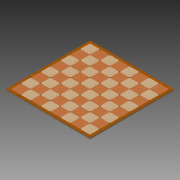
# Autodesk Inventor part: Spielfeld
Saved by Autodesk Inventor 2013 SP1 (Build 170176100, 176)
## iProperties
Created: 2012-12-06
Part Number: Spielfeld
Material: Esche
Document SubType Name: Modeling
Designer: Sebastian
Density: 1 g/cm^3
Author: Sebastian
Autodesk Inventor part; units mm, degrees
ref_plane "YZ Plane" through (0, 0, 0) normal (1, 0, 0) x (0, 1, 0)
ref_plane "XZ Plane" through (0, 0, 0) normal (0, 1, 0) x (-1, 0, 0)
ref_plane "XY Plane" through (0, 0, 0) normal (0, 0, 1) x (1, 0, 0)
sketch "Skizze5" plane through (0, 0, 0) normal (0, 0, 1) x (1, 0, 0)
  line L0 (0, 0) -> (40, 0)
  line L1 (40, 0) -> (40, 40)
  line L2 (40, 40) -> (0, 40)
  line L3 (0, 40) -> (0, 0)
  line L4 (40, 40) -> (80, 40)
  line L5 (80, 40) -> (80, 80)
  line L6 (80, 80) -> (40, 80)
  line L7 (40, 80) -> (40, 40)
  line L8 (80, 40) -> (120, 40)
  line L9 (120, 40) -> (120, 0)
  line L10 (120, 0) -> (80, 0)
  line L11 (80, 0) -> (80, 40)
  line L12 (120, 40) -> (160, 40)
  line L13 (160, 40) -> (160, 80)
  line L14 (160, 80) -> (120, 80)
  line L15 (120, 80) -> (120, 40)
  line L16 (0, 40) -> (-40, 40)
  line L17 (-40, 40) -> (-40, 80)
  line L18 (-40, 80) -> (0, 80)
  line L19 (0, 80) -> (0, 40)
  line L20 (-40, 40) -> (-80, 40)
  line L21 (-80, 40) -> (-80, 0)
  line L22 (-80, 0) -> (-40, 0)
  line L23 (-40, 0) -> (-40, 40)
  line L24 (-80, 40) -> (-120, 40)
  line L25 (-120, 40) -> (-120, 80)
  line L26 (-120, 80) -> (-80, 80)
  line L27 (-80, 80) -> (-80, 40)
  line L28 (-120, 40) -> (-160, 40)
  line L29 (-160, 40) -> (-160, 0)
  line L30 (-160, 0) -> (-120, 0)
  line L31 (-120, 0) -> (-120, 40)
  line L32 (0, 80) -> (40, 80)
  line L33 (40, 80) -> (40, 120)
  line L34 (40, 120) -> (0, 120)
  line L35 (0, 120) -> (0, 80)
  line L36 (40, 120) -> (80, 120)
  line L37 (80, 120) -> (80, 160)
  line L38 (80, 160) -> (40, 160)
  line L39 (40, 160) -> (40, 120)
  line L40 (80, 120) -> (120, 120)
  line L41 (120, 120) -> (120, 80)
  line L42 (120, 80) -> (80, 80)
  line L43 (80, 80) -> (80, 120)
  line L44 (120, 120) -> (160, 120)
  line L45 (160, 120) -> (160, 160)
  line L46 (160, 160) -> (120, 160)
  line L47 (120, 160) -> (120, 120)
  line L48 (0, 120) -> (-40, 120)
  line L49 (-40, 120) -> (-40, 160)
  line L50 (-40, 160) -> (0, 160)
  line L51 (0, 160) -> (0, 120)
  line L52 (-40, 120) -> (-80, 120)
  line L53 (-80, 120) -> (-80, 80)
  line L54 (-80, 80) -> (-40, 80)
  line L55 (-40, 80) -> (-40, 120)
  line L56 (-80, 120) -> (-120, 120)
  line L57 (-120, 120) -> (-120, 160)
  line L58 (-120, 160) -> (-80, 160)
  line L59 (-80, 160) -> (-80, 120)
  line L60 (-120, 120) -> (-160, 120)
  line L61 (-160, 120) -> (-160, 80)
  line L62 (-160, 80) -> (-120, 80)
  line L63 (-120, 80) -> (-120, 120)
  line L64 (0, -160) -> (40, -160)
  line L65 (40, -160) -> (40, -120)
  line L66 (40, -120) -> (0, -120)
  line L67 (0, -120) -> (0, -160)
  line L68 (40, -120) -> (80, -120)
  line L69 (80, -120) -> (80, -80)
  line L70 (80, -80) -> (40, -80)
  line L71 (40, -80) -> (40, -120)
  line L72 (80, -120) -> (120, -120)
  line L73 (120, -120) -> (120, -160)
  line L74 (120, -160) -> (80, -160)
  line L75 (80, -160) -> (80, -120)
  line L76 (120, -120) -> (160, -120)
  line L77 (160, -120) -> (160, -80)
  line L78 (160, -80) -> (120, -80)
  line L79 (120, -80) -> (120, -120)
  line L80 (0, -120) -> (-40, -120)
  line L81 (-40, -120) -> (-40, -80)
  line L82 (-40, -80) -> (0, -80)
  line L83 (0, -80) -> (0, -120)
  line L84 (-40, -120) -> (-80, -120)
  line L85 (-80, -120) -> (-80, -160)
  line L86 (-80, -160) -> (-40, -160)
  line L87 (-40, -160) -> (-40, -120)
  line L88 (-80, -120) -> (-120, -120)
  line L89 (-120, -120) -> (-120, -80)
  line L90 (-120, -80) -> (-80, -80)
  line L91 (-80, -80) -> (-80, -120)
  line L92 (-120, -120) -> (-160, -120)
  line L93 (-160, -120) -> (-160, -160)
  line L94 (-160, -160) -> (-120, -160)
  line L95 (-120, -160) -> (-120, -120)
  line L96 (-40, -80) -> (-40, -40)
  line L97 (-40, -40) -> (-40, 0)
  line L98 (-40, 0) -> (0, 0)
  line L99 (0, -40) -> (-40, -40)
  line L100 (0, 0) -> (0, -40)
  line L101 (0, -40) -> (0, -80)
  line L102 (40, 0) -> (40, -40)
  line L103 (40, -80) -> (40, -40)
  line L104 (0, -80) -> (40, -80)
  line L105 (80, 0) -> (40, 0)
  line L106 (40, -40) -> (80, -40)
  line L107 (40, -40) -> (0, -40)
  line L108 (-120, -40) -> (-160, -40)
  line L109 (-160, -40) -> (-160, -80)
  line L110 (-160, -80) -> (-120, -80)
  line L111 (-120, -80) -> (-120, -40)
  line L112 (-80, -40) -> (-80, -80)
  line L113 (-80, -80) -> (-40, -80)
  line L114 (-40, -40) -> (-80, -40)
  line L115 (-80, 0) -> (-80, -40)
  line L116 (-120, -40) -> (-120, 0)
  line L117 (-80, -40) -> (-120, -40)
  line L118 (-120, 0) -> (-80, 0)
  line L119 (160, -40) -> (160, 0)
  line L120 (120, -40) -> (160, -40)
  line L121 (120, -40) -> (120, -80)
  line L122 (120, 0) -> (120, -40)
  line L123 (120, -80) -> (80, -80)
  line L124 (80, -40) -> (120, -40)
  line L125 (80, -40) -> (80, 0)
  line L126 (80, -80) -> (80, -40)
  line L127 (160, 0) -> (120, 0)
  dimension "d639" = 40
  dimension "d640" = 40
  dimension "d641" = 40
  dimension "d642" = 40
  dimension "d643" = 40
  dimension "d644" = 40
  dimension "d645" = 40
  dimension "d646" = 40
  dimension "d647" = 40
  dimension "d648" = 40
  dimension "d649" = 40
  dimension "d650" = 40
  dimension "d651" = 40
  dimension "d652" = 40
  dimension "d653" = 40
  dimension "d654" = 40
  dimension "d655" = 40
  dimension "d656" = 40
  dimension "d657" = 40
  dimension "d658" = 40
  dimension "d659" = 40
  dimension "d660" = 40
  dimension "d661" = 40
  dimension "d662" = 40
  dimension "d663" = 40
  dimension "d664" = 40
  dimension "d665" = 40
  dimension "d666" = 40
  dimension "d667" = 40
  dimension "d668" = 40
  dimension "d669" = 40
  dimension "d670" = 40
  dimension "d671" = 40
  dimension "d672" = 40
  dimension "d673" = 40
  dimension "d674" = 40
  dimension "d675" = 40
  dimension "d676" = 40
  dimension "d677" = 40
  dimension "d678" = 40
  dimension "d679" = 40
  dimension "d680" = 40
  dimension "d681" = 40
  dimension "d682" = 40
  dimension "d683" = 40
  dimension "d684" = 40
  dimension "d685" = 40
  dimension "d686" = 40
  dimension "d687" = 40
  dimension "d688" = 40
  dimension "d689" = 40
  dimension "d690" = 40
  dimension "d691" = 40
  dimension "d692" = 40
  dimension "d693" = 40
  dimension "d694" = 40
  dimension "d695" = 40
  dimension "d696" = 40
  dimension "d697" = 40
  dimension "d698" = 40
  dimension "d699" = 40
  dimension "d700" = 40
  dimension "d701" = 40
  dimension "d702" = 40
  constraints: 256 end point, 64 parallel, 32 horizontal, 32 perpendicular
  measures "d639" distance of L2.end L1.end
  measures "d640" distance of L1.end L0.end
  measures "d641" distance of L6.end L5.end
  measures "d642" distance of L5.end L4.end
  measures "d643" distance of L9.end L10.end
  measures "d644" distance of L8.end L9.end
  measures "d645" distance of L14.end L13.end
  measures "d646" distance of L13.end L12.end
  measures "d647" distance of L17.end L18.end
  measures "d648" distance of L16.end L17.end
  measures "d649" distance of L22.end L21.end
  measures "d650" distance of L21.end L20.end
  measures "d651" distance of L25.end L26.end
  measures "d652" distance of L24.end L25.end
  measures "d653" distance of L30.end L29.end
  measures "d654" distance of L29.end L28.end
  measures "d655" distance of L48.start L39.end
  measures "d656" distance of L39.end L33.start
  measures "d657" distance of L39.start L38.start
  measures "d658" distance of L38.start L36.end
  measures "d659" distance of L41.end L42.end
  measures "d660" distance of L44.start L41.end
  measures "d661" distance of L47.start L45.end
  measures "d662" distance of L45.end L45.start
  measures "d663" distance of L49.end L50.end
  measures "d664" distance of L55.end L49.end
  measures "d665" distance of L55.start L53.end
  measures "d666" distance of L53.end L53.start
  measures "d667" distance of L57.end L59.start
  measures "d668" distance of L60.start L57.end
  measures "d669" distance of L62.end L61.end
  measures "d670" distance of L61.end L60.end
  measures "d671" distance of L66.end L66.start
  measures "d672" distance of L66.start L64.end
  measures "d673" distance of L71.start L70.start
  measures "d674" distance of L70.start L72.start
  measures "d675" distance of L74.start L74.end
  measures "d676" distance of L79.end L74.start
  measures "d677" distance of L79.start L77.end
  measures "d678" distance of L77.end L77.start
  measures "d679" distance of L81.end L82.end
  measures "d680" distance of L81.start L81.end
  measures "d681" distance of L87.start L86.start
  measures "d682" distance of L86.start L91.end
  measures "d683" distance of L90.start L90.end
  measures "d684" distance of L89.start L90.start
  measures "d685" distance of L95.start L94.start
  measures "d686" distance of L94.start L92.end
  measures "d687" distance of L99.start L107.start
  measures "d688" distance of L107.start L104.end
  measures "d689" distance of L102.start L105.start
  measures "d690" distance of L105.start L106.end
  measures "d691" distance of L123.start L123.end
  measures "d692" distance of L124.end L123.start
  measures "d693" distance of L122.start L119.end
  measures "d694" distance of L119.end L120.end
  measures "d695" distance of L97.end L98.end
  measures "d696" distance of L96.end L97.end
  measures "d697" distance of L96.start L113.start
  measures "d698" distance of L113.start L112.start
  measures "d699" distance of L116.end L115.start
  measures "d700" distance of L108.start L116.end
  measures "d701" distance of L110.end L110.start
  measures "d702" distance of L110.start L108.end
extrude "Extrusion Black" add sketch "Skizze5" against normal blind 1 contours L3 L2 L1 L0 | L100 L99 L97 L98 | L105 L125 L106 L102 | L16 L17 L18 L19 | L22 L21 L20 L23 | L107 L103 L104 L101 | L7 L6 L5 L4 | L11 L8 L9 L10 | L35 L34 L33 L32 | L115 L117 L116 L118 | L96 L113 L112 L114 | L83 L80 L81 L82 | L70 L69 L68 L71 | L124 L121 L123 L126 | L127 L119 L120 L122 | L95 L94 L93 L92 | L47 L46 L45 L44 | L54 L53 L52 L55 | L24 L25 L26 L27 | L48 L49 L50 L51 | L30 L29 L28 L31 | L66 L65 L64 L67 | L43 L40 L41 L42 | L15 L14 L13 L12 | L39 L38 L37 L36 | L91 L88 L89 L90 | L111 L110 L109 L108 | L87 L86 L85 L84 | L72 L73 L74 L75 | L78 L77 L76 L79 | L62 L61 L60 L63 | L56 L57 L58 L59
sketch "Skizze6" plane through (0, 0, 0) normal (0, 0, 1) x (1, 0, 0)
  line L0 (0, 0) -> (-40, 0)
  line L1 (-40, 0) -> (-40, 40)
  line L2 (-40, 40) -> (0, 40)
  line L3 (0, 40) -> (0, 0)
  line L4 (-40, 40) -> (-80, 40)
  line L5 (-80, 40) -> (-80, 80)
  line L6 (-80, 80) -> (-40, 80)
  line L7 (-40, 80) -> (-40, 40)
  line L8 (-80, 40) -> (-120, 40)
  line L9 (-120, 40) -> (-120, 0)
  line L10 (-120, 0) -> (-80, 0)
  line L11 (-80, 0) -> (-80, 40)
  line L12 (-120, 40) -> (-160, 40)
  line L13 (-160, 40) -> (-160, 80)
  line L14 (-160, 80) -> (-120, 80)
  line L15 (-120, 80) -> (-120, 40)
  line L16 (0, 40) -> (40, 40)
  line L17 (40, 40) -> (40, 80)
  line L18 (40, 80) -> (0, 80)
  line L19 (0, 80) -> (0, 40)
  line L20 (40, 40) -> (80, 40)
  line L21 (80, 40) -> (80, 0)
  line L22 (80, 0) -> (40, 0)
  line L23 (40, 0) -> (40, 40)
  line L24 (80, 40) -> (120, 40)
  line L25 (120, 40) -> (120, 80)
  line L26 (120, 80) -> (80, 80)
  line L27 (80, 80) -> (80, 40)
  line L28 (120, 40) -> (160, 40)
  line L29 (160, 40) -> (160, 0)
  line L30 (160, 0) -> (120, 0)
  line L31 (120, 0) -> (120, 40)
  line L32 (0, 80) -> (-40, 80)
  line L33 (-40, 80) -> (-40, 120)
  line L34 (-40, 120) -> (0, 120)
  line L35 (0, 120) -> (0, 80)
  line L36 (-40, 120) -> (-80, 120)
  line L37 (-80, 120) -> (-80, 160)
  line L38 (-80, 160) -> (-40, 160)
  line L39 (-40, 160) -> (-40, 120)
  line L40 (-80, 120) -> (-120, 120)
  line L41 (-120, 120) -> (-120, 80)
  line L42 (-120, 80) -> (-80, 80)
  line L43 (-80, 80) -> (-80, 120)
  line L44 (-120, 120) -> (-160, 120)
  line L45 (-160, 120) -> (-160, 160)
  line L46 (-160, 160) -> (-120, 160)
  line L47 (-120, 160) -> (-120, 120)
  line L48 (0, 120) -> (40, 120)
  line L49 (40, 120) -> (40, 160)
  line L50 (40, 160) -> (0, 160)
  line L51 (0, 160) -> (0, 120)
  line L52 (40, 120) -> (80, 120)
  line L53 (80, 120) -> (80, 80)
  line L54 (80, 80) -> (40, 80)
  line L55 (40, 80) -> (40, 120)
  line L56 (80, 120) -> (120, 120)
  line L57 (120, 120) -> (120, 160)
  line L58 (120, 160) -> (80, 160)
  line L59 (80, 160) -> (80, 120)
  line L60 (120, 120) -> (160, 120)
  line L61 (160, 120) -> (160, 80)
  line L62 (160, 80) -> (120, 80)
  line L63 (120, 80) -> (120, 120)
  line L64 (0, -160) -> (-40, -160)
  line L65 (-40, -160) -> (-40, -120)
  line L66 (-40, -120) -> (0, -120)
  line L67 (0, -120) -> (0, -160)
  line L68 (-40, -120) -> (-80, -120)
  line L69 (-80, -120) -> (-80, -80)
  line L70 (-80, -80) -> (-40, -80)
  line L71 (-40, -80) -> (-40, -120)
  line L72 (-80, -120) -> (-120, -120)
  line L73 (-120, -120) -> (-120, -160)
  line L74 (-120, -160) -> (-80, -160)
  line L75 (-80, -160) -> (-80, -120)
  line L76 (-120, -120) -> (-160, -120)
  line L77 (-160, -120) -> (-160, -80)
  line L78 (-160, -80) -> (-120, -80)
  line L79 (-120, -80) -> (-120, -120)
  line L80 (0, -120) -> (40, -120)
  line L81 (40, -120) -> (40, -80)
  line L82 (40, -80) -> (0, -80)
  line L83 (0, -80) -> (0, -120)
  line L84 (40, -120) -> (80, -120)
  line L85 (80, -120) -> (80, -160)
  line L86 (80, -160) -> (40, -160)
  line L87 (40, -160) -> (40, -120)
  line L88 (80, -120) -> (120, -120)
  line L89 (120, -120) -> (120, -80)
  line L90 (120, -80) -> (80, -80)
  line L91 (80, -80) -> (80, -120)
  line L92 (120, -120) -> (160, -120)
  line L93 (160, -120) -> (160, -160)
  line L94 (160, -160) -> (120, -160)
  line L95 (120, -160) -> (120, -120)
  line L96 (120, -40) -> (160, -40)
  line L97 (80, -40) -> (120, -40)
  line L98 (120, 0) -> (80, 0)
  line L99 (120, -40) -> (120, 0)
  line L100 (120, -80) -> (120, -40)
  line L101 (160, -40) -> (160, -80)
  line L102 (160, -80) -> (120, -80)
  line L103 (80, 0) -> (80, -40)
  line L104 (80, -40) -> (80, -80)
  line L105 (80, -80) -> (40, -80)
  line L106 (40, -40) -> (80, -40)
  line L107 (40, -80) -> (40, -40)
  line L108 (0, -40) -> (0, -80)
  line L109 (40, -40) -> (40, 0)
  line L110 (0, -40) -> (40, -40)
  line L111 (0, 0) -> (0, -40)
  line L112 (40, 0) -> (0, 0)
  line L113 (-80, -40) -> (-120, -40)
  line L114 (-120, -80) -> (-80, -80)
  line L115 (-120, -40) -> (-120, -80)
  line L116 (-120, -40) -> (-160, -40)
  line L117 (-160, 0) -> (-120, 0)
  line L118 (-160, -40) -> (-160, 0)
  line L119 (-120, 0) -> (-120, -40)
  line L120 (-40, -40) -> (0, -40)
  line L121 (0, -80) -> (-40, -80)
  line L122 (-40, 0) -> (-40, -40)
  line L123 (-40, -80) -> (-40, -40)
  line L124 (-80, -40) -> (-80, 0)
  line L125 (-80, 0) -> (-40, 0)
  line L126 (-40, -40) -> (-80, -40)
  line L127 (-80, -80) -> (-80, -40)
  dimension "d703" = 40
  dimension "d704" = 40
  dimension "d705" = 40
  dimension "d706" = 40
  dimension "d707" = 40
  dimension "d708" = 40
  dimension "d709" = 40
  dimension "d710" = 40
  dimension "d711" = 40
  dimension "d712" = 40
  dimension "d713" = 40
  dimension "d714" = 40
  dimension "d715" = 40
  dimension "d716" = 40
  dimension "d717" = 40
  dimension "d718" = 40
  dimension "d719" = 40
  dimension "d720" = 40
  dimension "d721" = 40
  dimension "d722" = 40
  dimension "d723" = 40
  dimension "d724" = 40
  dimension "d725" = 40
  dimension "d726" = 40
  dimension "d727" = 40
  dimension "d728" = 40
  dimension "d729" = 40
  dimension "d730" = 40
  dimension "d731" = 40
  dimension "d732" = 40
  dimension "d733" = 40
  dimension "d734" = 40
  dimension "d735" = 40
  dimension "d736" = 40
  dimension "d737" = 40
  dimension "d738" = 40
  dimension "d739" = 40
  dimension "d740" = 40
  dimension "d741" = 40
  dimension "d742" = 40
  dimension "d743" = 40
  dimension "d744" = 40
  dimension "d745" = 40
  dimension "d746" = 40
  dimension "d747" = 40
  dimension "d748" = 40
  dimension "d749" = 40
  dimension "d750" = 40
  dimension "d751" = 40
  dimension "d752" = 40
  dimension "d753" = 40
  dimension "d754" = 40
  dimension "d755" = 40
  dimension "d756" = 40
  dimension "d757" = 40
  dimension "d758" = 40
  dimension "d759" = 40
  dimension "d760" = 40
  dimension "d761" = 40
  dimension "d762" = 40
  dimension "d763" = 40
  dimension "d764" = 40
  dimension "d765" = 40
  dimension "d766" = 40
  constraints: 256 end point, 64 parallel, 32 horizontal, 32 perpendicular
  measures "d703" distance of L1.end L2.end
  measures "d704" distance of L0.end L1.end
  measures "d705" distance of L5.end L6.end
  measures "d706" distance of L4.end L5.end
  measures "d707" distance of L10.end L9.end
  measures "d708" distance of L9.end L8.end
  measures "d709" distance of L13.end L14.end
  measures "d710" distance of L12.end L13.end
  measures "d711" distance of L18.end L17.end
  measures "d712" distance of L17.end L16.end
  measures "d713" distance of L21.end L22.end
  measures "d714" distance of L20.end L21.end
  measures "d715" distance of L26.end L25.end
  measures "d716" distance of L25.end L24.end
  measures "d717" distance of L29.end L30.end
  measures "d718" distance of L28.end L29.end
  measures "d719" distance of L34.start L35.start
  measures "d720" distance of L32.end L34.start
  measures "d721" distance of L37.end L39.start
  measures "d722" distance of L40.start L37.end
  measures "d723" distance of L42.end L42.start
  measures "d724" distance of L42.start L40.end
  measures "d725" distance of L46.start L46.end
  measures "d726" distance of L44.end L46.start
  measures "d727" distance of L51.start L49.end
  measures "d728" distance of L49.end L52.start
  measures "d729" distance of L53.end L54.end
  measures "d730" distance of L56.start L53.end
  measures "d731" distance of L58.end L58.start
  measures "d732" distance of L58.start L60.start
  measures "d733" distance of L61.end L63.start
  measures "d734" distance of L60.end L61.end
  measures "d735" distance of L68.start L83.end
  measures "d736" distance of L65.start L68.start
  measures "d737" distance of L69.end L70.end
  measures "d738" distance of L69.start L69.end
  measures "d739" distance of L74.end L73.end
  measures "d740" distance of L73.end L72.end
  measures "d741" distance of L77.end L79.start
  measures "d742" distance of L76.end L77.end
  measures "d743" distance of L82.end L81.end
  measures "d744" distance of L81.end L84.start
  measures "d745" distance of L86.start L87.start
  measures "d746" distance of L84.end L86.start
  measures "d747" distance of L91.start L89.end
  measures "d748" distance of L89.end L88.end
  measures "d749" distance of L93.end L95.start
  measures "d750" distance of L92.end L93.end
  measures "d751" distance of L122.end L110.start
  measures "d752" distance of L123.start L122.end
  measures "d753" distance of L124.end L122.start
  measures "d754" distance of L113.start L124.end
  measures "d755" distance of L114.end L115.end
  measures "d756" distance of L115.end L113.end
  measures "d757" distance of L117.start L119.start
  measures "d758" distance of L116.end L117.start
  measures "d759" distance of L111.start L109.end
  measures "d760" distance of L109.end L110.end
  measures "d761" distance of L105.start L105.end
  measures "d762" distance of L97.start L105.start
  measures "d763" distance of L103.start L99.end
  measures "d764" distance of L99.end L97.end
  measures "d765" distance of L102.start L102.end
  measures "d766" distance of L96.end L102.start
extrude "Extrusion White" add sketch "Skizze6" against normal blind 1 separate body contours L0 L1 L2 L3 | L112 L109 L110 L111 | L122 L126 L124 L125 | L19 L18 L17 L16 | L108 L121 L123 L120 | L23 L20 L21 L22 | L4 L5 L6 L7 | L10 L9 L8 L11 | L32 L33 L34 L35 | L82 L81 L80 L83 | L106 L104 L105 L107 | L98 L99 L97 L103 | L71 L68 L69 L70 | L127 L114 L115 L113 | L44 L45 L46 L47 | L92 L93 L94 L95 | L119 L116 L118 L117 | L55 L52 L53 L54 | L27 L26 L25 L24 | L51 L50 L49 L48 | L67 L64 L65 L66 | L31 L28 L29 L30 | L42 L41 L40 L43 | L12 L13 L14 L15 | L36 L37 L38 L39 | L84 L85 L86 L87 | L90 L89 L88 L91 | L96 L101 L102 L100 | L75 L74 L73 L72 | L79 L76 L77 L78 | L63 L60 L61 L62 | L59 L58 L57 L56
sketch "Skizze7" plane through (0, 0, 0) normal (0, 0, 1) x (1, 0, 0)
  line L0 (-170, -170) -> (170, -170)
  line L1 (-170, -170) -> (-160, -160)
  line L2 (-160, -160) -> (160, -160)
  line L3 (160, -160) -> (170, -170)
  point P0 (0, 0)
  dimension "d599" = 340
  constraints: 8 end point, 1 horizontal, 1 perpendicular
  measures "d599" distance of L0.start L0.end
extrude "Extrusion Kachelleiste unten" add sketch "Skizze7" against normal blind 1 separate body
sketch "Skizze8" plane through (0, 0, 0) normal (0, 0, 1) x (1, 0, 0)
  line L0 (-170, -170) -> (-170, 170)
  line L1 (-170, 170) -> (-160, 160)
  line L2 (-160, 160) -> (-160, -160)
  line L3 (-160, -160) -> (-170, -170)
  point P0 (0, 0)
  dimension "d603" = 340
  constraints: 8 end point, 1 parallel, 1 perpendicular, 1 vertical
  measures "d603" distance of L0.start L0.end
extrude "Extrusion Kachelleiste links" add sketch "Skizze8" against normal blind 1 separate body
sketch "Skizze9" plane through (0, 0, 0) normal (0, 0, 1) x (1, 0, 0)
  line L0 (-170, 170) -> (170, 170)
  line L1 (160, 160) -> (170, 170)
  line L2 (160, 160) -> (-160, 160)
  line L3 (-160, 160) -> (-170, 170)
  point P0 (0, 0)
  dimension "d606" = 340
  constraints: 8 end point, 1 horizontal, 1 parallel, 1 perpendicular
  measures "d606" distance of L0.start L0.end
extrude "Extrusion Kachelleiste oben" add sketch "Skizze9" against normal blind 1 separate body
sketch "Skizze10" plane through (0, 0, 0) normal (0, 0, 1) x (1, 0, 0)
  line L0 (170, -170) -> (170, 170)
  line L1 (160, -160) -> (170, -170)
  line L2 (160, -160) -> (160, 160)
  line L3 (160, 160) -> (170, 170)
  point P0 (0, 0)
  dimension "d609" = 340
  dimension "d610" = 320
  constraints: 8 end point, 1 parallel, 1 perpendicular, 1 vertical
  measures "d609" distance of L0.start L0.end
  measures "d610" distance of L1.start L2.end
extrude "Extrusion Kachelleiste rechts" add sketch "Skizze10" against normal blind 1 separate body
hole "Bohrung2" at (-160, -160, 0) direction (0, 0, -1) diameter 5 depth 12 tip angle 118 bodies 1
pattern_linear "Rechteckige Anordnung1" count 9 spacing 40 along (0, 1, 0) count 9 spacing 40 along (1, 0, 0) of "Bohrung2" bodies 1
hole "Bohrung3" at (-160, 160, 0) direction (0, 0, -1) diameter 5 depth 12 tip angle 118 bodies 2
pattern_linear "Rechteckige Anordnung2" count 9 spacing 40 along (1, 0, 0) count 9 spacing 40 along (0, -1, 0) of "Bohrung3" bodies 2
hole "Bohrung4" at (-160, 160, 0) direction (0, 0, -1) diameter 5 depth 12 tip angle 118 bodies 5
pattern_linear "Rechteckige Anordnung3" count 9 spacing 40 along (1, 0, 0) of "Bohrung4" bodies 5
hole "Bohrung5" at (160, 160, 0) direction (0, 0, -1) diameter 5 depth 12 tip angle 118 bodies 6
pattern_linear "Rechteckige Anordnung4" count 9 spacing 40 along (0, -1, 0) of "Bohrung5" bodies 6
hole "Bohrung6" at (160, -160, 0) direction (0, 0, -1) diameter 5 depth 12 tip angle 118 bodies 3
pattern_linear "Rechteckige Anordnung5" count 9 spacing 40 along (-1, 0, 0) of "Bohrung6" bodies 3
hole "Bohrung7" at (-160, -160, 0) direction (0, 0, -1) diameter 5 depth 12 tip angle 118 bodies 4
pattern_linear "Rechteckige Anordnung6" count 9 spacing 40 along (0, 1, 0) of "Bohrung7" bodies 4
sketch "Skizze17" plane through (0, 0, 0) normal (0, 0, 1) x (1, 0, 0)
  line L0 (-170, -170) -> (170, -170)
  line L1 (170, -170) -> (170, 170)
  line L2 (170, 170) -> (-170, 170)
  line L3 (-170, 170) -> (-170, -170)
  point P0 (0, 0)
  constraints: 8 end point, 2 parallel, 1 horizontal, 1 perpendicular
extrude "Extrusion Boden" add sketch "Skizze17" against normal blind 6 separate body
move or copy body "Körper verschieben Boden" bodies to move or copy 7 copy no translate (0, 0, -1)
hole "Bohrung Boden" at (-160, 160, -1) direction (0, 0, -1) diameter 5 depth 12 tip angle 118 bodies 7
pattern_linear "Rechteckige Anordnung7" count 9 spacing 40 along (1, 0, 0) count 9 spacing 40 along (0, -1, 0) of "Bohrung Boden" bodies 7
